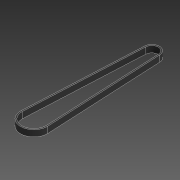
# Autodesk Inventor part: tandriem32Tnaar16T_lengte280
Saved by Autodesk Inventor 2020 (Build 240168000, 168)
## iProperties
Created: 2020-05-15
Part Number: tandriem32Tnaar16T_lengte280
Material: Generic
Document SubType Name: Modeling
Designer: stefa
Density: 1 g/cm^3
Appearance: Rubber - Black
Author: stefa
Autodesk Inventor part; units mm, degrees
ref_plane "YZ Plane" through (0, 0, 0) normal (1, 0, 0) x (0, 1, 0)
ref_plane "XZ Plane" through (0, 0, 0) normal (0, 1, 0) x (-1, 0, 0)
ref_plane "XY Plane" through (0, 0, 0) normal (0, 0, 1) x (1, 0, 0)
sketch "Sketch1" plane through (0, 0, 0) normal (0, 1, 0) x (-1, 0, 0)
  arc A0 (11.4863, -0.5615) -> (-11.4863, -0.5615) centre (0, 0) ccw
  arc A1 (-5.9928, -112.9383) -> (5.9928, -112.9383) centre (0, -112.6454) ccw
  line L0 (11.4863, -0.5615) -> (5.9928, -112.9383)
  line L1 (-5.9928, -112.9383) -> (-11.4863, -0.5615)
  line L2 (7.2913, -113.0018) -> (12.7847, -0.625)
  arc A2 (12.7847, -0.625) -> (-12.7847, -0.625) centre (0, 0) ccw
  line L3 (-12.7847, -0.625) -> (-7.2913, -113.0018)
  arc A3 (-7.2913, -113.0018) -> (7.2913, -113.0018) centre (0, -112.6454) ccw
  dimension "d0" = 23
  dimension "d1" = 12
  dimension "d2" = 112.511
  dimension "d6" = 1.3
  constraints: 8 end point, 8 point on circle, 4 centre point, 3 tangent, 1 coincident, 1 equal length, 1 vertical alignment, 3 other
  measures "d0" diameter of A0
  measures "d1" diameter of A1
  measures "d2" distance of L0.start L0.end
  measures "d6" distance between parallel lines of L0 L2
extrude "Extrusion1" add sketch "Sketch1" along normal blind 6
body "Solid1"
